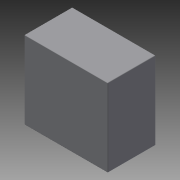
# Autodesk Inventor part: PSU
Saved by Autodesk Inventor 2015 (Build 190159000, 159)
## iProperties
Created: 2016-03-23
Part Number: PSU
Material: Generic
Document SubType Name: Modeling
Designer: Noah
Density: 1 g/cm^3
Appearance: Default
Author: Noah
Autodesk Inventor part; units mm, degrees
ref_plane "YZ Plane" through (0, 0, 0) normal (1, 0, 0) x (0, 1, 0)
ref_plane "XZ Plane" through (0, 0, 0) normal (0, 1, 0) x (-1, 0, 0)
ref_plane "XY Plane" through (0, 0, 0) normal (0, 0, 1) x (1, 0, 0)
sketch "Sketch1" plane through (0, 0, 0) normal (0, 1, 0) x (-1, 0, 0)
  line L0 (-75, -70) -> (75, -70)
  line L1 (75, -70) -> (75, 70)
  line L2 (75, 70) -> (-75, 70)
  line L3 (-75, 70) -> (-75, -70)
  point P0 (0, 0)
  dimension "d0" = 150
  dimension "d1" = 140
  dimension "d4" = 70
  dimension "d5" = 75
  constraints: 8 end point, 2 parallel, 1 horizontal, 1 perpendicular
  measures "d0" distance of L0.start L0.end
  measures "d1" distance of L0.end L1.end
  measures "d4" distance from line of point (0, 0) L0
  measures "d5" distance from line of L1 point (0, 0)
extrude "Extrusion1" add sketch "Sketch1" along normal blind 86
fillet "Fillet1" radius 1 12 edges at (0, 0, 70) (-75, 43, 70) (-75, 86, 0) (-75, 0, 0) (-75, 43, -70) (75, 43, 70) (0, 86, 70) (75, 86, 0) (75, 43, -70) (0, 86, -70) (0, 0, -70) (75, 0, 0)
body "Solid1"
